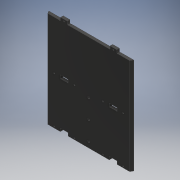
# Autodesk Inventor part: BA04
Saved by Autodesk Inventor 2017 (Build 210142000, 142)
## iProperties
Created: 2019-05-22
Part Number: BA04
Material: Wood (Cherry)
Document SubType Name: Modeling
Designer: Dell
Density: 0.63 g/cm^3
Appearance: Smooth - Black
Mass: 794.992 g
Surface Area: 2256.82 cm^2
Volume: 1261.89 cm^3
Author: Dell
Autodesk Inventor part; units mm, degrees
ref_plane "YZ Plane" through (0, 0, 0) normal (1, 0, 0) x (0, 1, 0)
ref_plane "XZ Plane" through (0, 0, 0) normal (0, 1, 0) x (-1, 0, 0)
ref_plane "XY Plane" through (0, 0, 0) normal (0, 0, 1) x (1, 0, 0)
sketch "Sketch1" plane through (0, 0, 0) normal (0, 0, 1) x (1, 0, 0)
  line L0 (0, 0) -> (303.5592, 0)
  line L1 (303.5592, 0) -> (455.3388, -262.89) construction
  line L2 (455.3388, -262.89) -> (404.5388, -350.8782)
  line L3 (404.5388, -350.8782) -> (-50.8, -87.9882) construction
  line L4 (-50.8, -87.9882) -> (0, 0) construction
  line L5 (0, 0) -> (5.4993, -9.525)
  line L6 (5.4993, -9.525) -> (298.06, -9.525)
  line L7 (298.06, -9.525) -> (303.5592, 0)
  dimension "d0" = 525.78
  dimension "d1" = 101.6
  dimension "d2" = 120
  dimension "d3" = 9.525
  dimension "d4" = 60
  dimension "d5" = 60
  constraints: 16 end point, 2 equal length, 2 horizontal, 2 perpendicular
  measures "d0" distance of L2.end L3.end
  measures "d1" distance of L3.end L0.start
  measures "d2" angle of L0 L4
  measures "d3" distance between parallel lines of L0 L6
  measures "d4" angle of L0 L5
  measures "d5" angle of L0 L7
extrude "Extrusion1" add sketch "Sketch1" along normal blind 342.9
sketch "Sketch2" plane through (5.4993, -9.525, 0) normal (0, -1, 0) x (1, 0, 0)
  line L0 (298.06, 342.9) -> (-5.4993, 342.9) projected
  line L1 (45.3007, 342.9) -> (70.7007, 342.9)
  line L2 (70.7007, 342.9) -> (70.7007, 352.425)
  line L3 (70.7007, 352.425) -> (45.3007, 352.425)
  line L4 (45.3007, 352.425) -> (45.3007, 342.9)
  line L5 (221.86, 342.9) -> (247.26, 342.9)
  line L6 (247.26, 342.9) -> (247.26, 352.425)
  line L7 (247.26, 352.425) -> (221.86, 352.425)
  line L8 (221.86, 352.425) -> (221.86, 342.9)
  line L9 (-5.4993, 0) -> (-5.4993, 342.9) projected
  line L10 (298.06, 0) -> (298.06, 342.9) projected
  circle A0 centre (58.0007, 347.6625) radius 2.25
  circle A1 centre (234.56, 347.6625) radius 2.25
  point P0 (58.0007, 352.425)
  point P1 (234.56, 352.425)
  point P2 (70.7007, 347.6625)
  point P3 (247.26, 347.6625)
  dimension "d8" = 25.4
  dimension "d9" = 9.525
  dimension "d10" = 25.4
  dimension "d11" = 9.525
  dimension "d12" = 50.8
  dimension "d13" = 50.8
  dimension "d16" = 4.5
  dimension "d17" = 4.5
  constraints: 16 end point, 4 midpoint, 4 parallel, 2 centre point, 2 horizontal, 2 horizontal alignment, 2 perpendicular, 2 point on line, 2 vertical alignment
  measures "d8" distance of L3.end L2.end
  measures "d9" distance of L2.end L1.end
  measures "d10" distance of L7.end L6.end
  measures "d11" distance of L6.end L5.end
  measures "d12" distance between parallel lines of L9 L4
  measures "d13" distance between parallel lines of L10 L6
  measures "d16" diameter of A0
  measures "d17" diameter of A1
extrude "Extrusion2" add sketch "Sketch2" against normal blind 9.525
ref_plane "Work Plane1" through (0, 0, 292.1) normal (0, 0, 1) x (1, 0, 0)
sketch "Sketch3" plane through (0, 0, 292.1) normal (0, 0, 1) x (1, 0, 0)
  line L0 (0, 0) -> (303.5592, 0) projected
  line L1 (0, 0) -> (0, -9.525)
  line L2 (298.06, -9.525) -> (5.4993, -9.525) projected
  line L3 (0, -9.525) -> (5.4993, -9.525)
  line L4 (5.4993, -9.525) -> (0, 0) projected
  constraints: 4 end point, 1 perpendicular, 1 vertical
extrude "Extrusion3" [suppressed]
ref_plane "Work Plane2" through (0, 0, 50.8) normal (0, 0, -1) x (-1, 0, 0)
sketch "Sketch4" plane through (0, 0, 50.8) normal (0, 0, -1) x (-1, 0, 0)
  line L0 (0, -12.7) -> (0, 0) projected
  line L1 (-7.3323, -12.7) -> (0, 0) projected
  line L2 (-7.3323, -12.7) -> (0, -12.7) projected
extrude "Extrusion4" [suppressed]
ref_plane "Work Plane3" through (0, 0, 171.45) normal (0, 0, -1) x (-1, 0, 0)
sketch "Sketch5" plane through (0, 0, 171.45) normal (0, 0, -1) x (-1, 0, 0)
  line L0 (0, 0) -> (0, -12.7) projected
  line L1 (0, -12.7) -> (-7.3323, -12.7) projected
  line L2 (0, 0) -> (-7.3323, -12.7) projected
extrude "Extrusion5" [suppressed]
ref_plane "Work Plane4" through (151.7796, -9.525, 342.9) normal (-1, 0, 0) x (0, 0, 1)
mirror "Mirror1" [suppressed]
sketch "Sketch6" plane through (296.2269, -12.7, 292.1) normal (0, 0, 1) x (1, 0, 0)
  line L0 (0, 0) -> (7.3323, 12.7) projected
  line L1 (7.3323, 0) -> (0, 0) projected
  line L2 (7.3323, 12.7) -> (7.3323, 0) projected
  line L3 (7.3323, 12.7) -> (7.3323, 0) projected
  line L4 (0, 0) -> (7.3323, 12.7) projected
  line L5 (7.3323, 0) -> (0, 0) projected
  line L6 (-296.2269, 12.7) -> (-296.2269, 0) projected
  line L7 (-296.2269, 0) -> (-288.8945, 0) projected
  line L8 (-296.2269, 12.7) -> (-288.8945, 0) projected
  line L9 (-296.2269, 0) -> (-296.2269, 12.7) projected
  line L10 (-296.2269, 12.7) -> (-274.2298, 0) construction
  line L11 (0, 0) -> (-288.8945, 0) projected
  line L12 (-285.2269, 6.3491) -> (-285.2269, 0)
  line L13 (-288.8945, 0) -> (-296.2269, 0) projected
  line L14 (-285.2269, 0) -> (-296.2269, 0)
  line L15 (-144.4473, 0) -> (-144.4473, -42.8761)
  line L16 (7.3323, 12.7) -> (7.3323, 0)
  line L17 (7.3323, 0) -> (0, 0)
  line L18 (7.3323, 12.7) -> (0, 0)
  line L19 (7.3323, 0) -> (7.3323, 12.7)
  line L20 (7.3323, 12.7) -> (-14.6647, 0) construction
  line L21 (-3.6677, 6.3491) -> (-3.6677, 0)
  line L22 (0, 0) -> (7.3323, 0)
  line L23 (-3.6677, 0) -> (7.3323, 0)
  line L24 (-288.8945, 0) -> (-296.2269, 12.7) projected
  line L25 (-285.2269, 6.3491) -> (-296.2269, 12.7)
  line L26 (7.3323, 12.7) -> (0, 0) projected
  line L27 (7.3323, 12.7) -> (-3.6677, 6.3491)
  line L28 (0, 0) -> (7.3323, 12.7)
  line L29 (0, 0) -> (-3.6677, 0)
  line L30 (7.3323, 0) -> (7.3323, 12.7) projected
  line L31 (-3.6677, 0) -> (7.3323, 0)
  dimension "d26" = 60
  dimension "d27" = 11
  constraints: 34 end point, 5 symmetric about line, 3 point on line, 2 collinear, 2 horizontal, 1 midpoint, 1 perpendicular, 1 vertical
  measures "d26" angle of L6 L10
  measures "d27" distance between parallel lines of L6 L12
extrude "Extrusion6" [suppressed]
sketch "Sketch7" plane through (0, 0, 184.15) normal (0, 0, 1) x (1, 0, 0)
  line L0 (7.3323, -12.7) -> (0, 0) projected
  line L1 (11, -12.7) -> (7.3323, -12.7) projected
  line L2 (11, -6.3509) -> (11, -12.7) projected
  line L3 (0, 0) -> (11, -6.3509) projected
  line L4 (303.5592, 0) -> (296.2269, -12.7) projected
  line L5 (292.5592, -6.3509) -> (303.5592, 0) projected
  line L6 (292.5592, -12.7) -> (292.5592, -6.3509) projected
  line L7 (296.2269, -12.7) -> (292.5592, -12.7) projected
  line L8 (303.5592, 0) -> (303.5592, -12.7) projected
  line L9 (296.2269, -12.7) -> (303.5592, 0) projected
  line L10 (303.5592, -12.7) -> (296.2269, -12.7) projected
  line L11 (0, 0) -> (0, -12.7) projected
  line L12 (0, -12.7) -> (7.3323, -12.7) projected
  line L13 (0, 0) -> (7.3323, -12.7) projected
extrude "Extrusion7" [suppressed]
sketch "Sketch8" plane through (0, 0, 76.2) normal (0, 0, 1) x (1, 0, 0)
  line L0 (0, 0) -> (0, -12.7) projected
  line L1 (0, -12.7) -> (7.3323, -12.7) projected
  line L2 (0, 0) -> (7.3323, -12.7) projected
  line L3 (7.3323, -12.7) -> (0, 0) projected
  line L4 (11, -12.7) -> (7.3323, -12.7) projected
  line L5 (11, -6.3509) -> (11, -12.7) projected
  line L6 (0, 0) -> (11, -6.3509) projected
  line L7 (303.5592, 0) -> (296.2269, -12.7) projected
  line L8 (292.5592, -6.3509) -> (303.5592, 0) projected
  line L9 (292.5592, -12.7) -> (292.5592, -6.3509) projected
  line L10 (296.2269, -12.7) -> (292.5592, -12.7) projected
  line L11 (303.5592, 0) -> (303.5592, -12.7) projected
  line L12 (296.2269, -12.7) -> (303.5592, 0) projected
  line L13 (303.5592, -12.7) -> (296.2269, -12.7) projected
extrude "Extrusion8" [suppressed]
sketch "Sketch9" plane through (0, 0, 0) normal (0, 0, -1) x (-1, 0, 0)
  line L0 (-251.9796, -9.525) -> (-251.9796, 0)
  line L1 (-251.9796, 0) -> (-226.5796, 0)
  line L2 (-226.5796, 0) -> (-226.5796, -9.525)
  line L3 (-226.5796, -9.525) -> (-251.9796, -9.525)
  line L4 (-76.9796, -9.525) -> (-76.9796, 0)
  line L5 (-76.9796, 0) -> (-51.5796, 0)
  line L6 (-51.5796, 0) -> (-51.5796, -9.525)
  line L7 (-51.5796, -9.525) -> (-76.9796, -9.525)
  line L8 (-239.2796, 0) -> (-64.2796, 0) construction
  circle A0 centre (-239.2796, -4.7625) radius 2.25
  circle A1 centre (-64.2796, -4.7625) radius 2.25
  line L9 (-239.2796, -4.7625) -> (-239.2796, 0) construction
  line L10 (-239.2796, -4.7625) -> (-226.5796, -4.7625) construction
  line L11 (-76.9796, -4.7625) -> (-64.2796, -4.7625) construction
  line L12 (-64.2796, -4.7625) -> (-64.2796, 0) construction
  line L13 (0, 0) -> (-303.5592, 0) projected
  point P0 (-151.7796, 0)
  dimension "d34" = 25.4
  dimension "d35" = 9.525
  dimension "d36" = 9.525
  dimension "d37" = 25.4
  dimension "d38" = 175
  dimension "d39" = 4.5
  dimension "d40" = 4.5
  constraints: 26 end point, 6 midpoint, 6 perpendicular, 4 parallel, 4 point on line, 2 centre point
  measures "d34" distance of L4.end L5.end
  measures "d35" distance of L5.end L7.start
  measures "d36" distance of L0.start L1.start
  measures "d37" distance of L1.start L2.start
  measures "d38" distance of L8.start L12.end
  measures "d39" diameter of A0
  measures "d40" diameter of A1
extrude "Extrusion9" cut sketch "Sketch9" against normal blind 9.525 contours L0 L1 L2 L3 | L4 L5 L6 L7 | A0 | A1
sketch "Sketch10" plane through (227.3592, -9.525, 352.425) normal (0, -1, 0) x (1, 0, 0)
  line L0 (-175.7796, -187.8) -> (-150.3796, -187.8)
  line L1 (-150.3796, -187.8) -> (-150.3796, -178.275)
  line L2 (-150.3796, -178.275) -> (-175.7796, -178.275)
  line L3 (-175.7796, -178.275) -> (-175.7796, -187.8)
  line L4 (-0.7796, -187.8) -> (24.6204, -187.8)
  line L5 (24.6204, -187.8) -> (24.6204, -178.275)
  line L6 (24.6204, -178.275) -> (-0.7796, -178.275)
  line L7 (-0.7796, -178.275) -> (-0.7796, -187.8)
  line L8 (-175.7796, -342.9) -> (-150.3796, -342.9) projected
  line L9 (-0.7796, -342.9) -> (24.6204, -342.9) projected
  line L10 (76.2, -9.525) -> (-227.3592, -9.525) projected
  point P0 (-227.3592, -352.425)
  point P1 (-163.0796, -187.8)
  point P2 (-163.0796, -342.9)
  point P3 (11.9204, -187.8)
  point P4 (11.9204, -342.9)
  point P5 (-176.5592, -9.525)
  dimension "d44" = 25.4
  dimension "d45" = 9.525
  dimension "d46" = 25.4
  dimension "d47" = 9.525
  dimension "d90" = 168.75
  constraints: 16 end point, 4 midpoint, 4 parallel, 2 horizontal, 2 perpendicular, 2 vertical alignment, 1 horizontal alignment
  measures "d44" distance of L2.end L1.end
  measures "d45" distance of L1.end L0.end
  measures "d46" distance of L6.end L5.end
  measures "d47" distance of L5.end L4.end
  measures "d90" distance between parallel lines of L10 L2
extrude "Extrusion10" cut sketch "Sketch10" against normal through all
sketch "Sketch11" plane through (227.3592, -9.525, 352.425) normal (0, -1, 0) x (1, 0, 0)
  line L0 (-150.3796, -352.425) -> (-0.7796, -352.425) construction
  line L1 (-100.9796, -352.425) -> (-50.1796, -352.425) construction
  line L2 (-50.1796, -352.425) -> (-50.1796, -178.275) construction
  line L3 (-50.1796, -178.275) -> (-100.9796, -178.275) construction
  line L4 (-100.9796, -178.275) -> (-100.9796, -352.425) construction
  circle A0 centre (-75.5796, -264.715) radius 4
  circle A1 centre (-75.5796, -197.005) radius 4
  circle A2 centre (-75.5796, -332.425) radius 4
  line L5 (-0.7796, -352.425) -> (-150.3796, -352.425) projected
  circle A3 centre (-198.8198, -183.0375) radius 2.25
  circle A4 centre (-198.8198, -347.6625) radius 2.25
  circle A5 centre (47.6606, -347.6625) radius 2.25
  circle A6 centre (47.6606, -183.0375) radius 2.25
  line L6 (-175.7796, -352.425) -> (-221.86, -352.425) projected
  line L7 (70.7007, -352.425) -> (24.6204, -352.425) projected
  line L8 (-175.7796, -187.8) -> (-175.7796, -178.275) projected
  line L9 (-175.7796, -352.425) -> (-175.7796, -342.9) projected
  line L10 (24.6204, -342.9) -> (24.6204, -352.425) projected
  line L11 (24.6204, -178.275) -> (24.6204, -187.8) projected
  circle A7 centre (-126.3796, -183.0375) radius 2.25
  circle A8 centre (-126.3796, -347.6625) radius 2.25
  circle A9 centre (-24.7796, -347.6625) radius 2.25
  circle A10 centre (-24.7796, -183.0375) radius 2.25
  point P0 (-227.3592, -352.425)
  point P1 (-150.3796, -178.275)
  point P2 (-75.5796, -352.425)
  point P3 (-75.5796, -352.425)
  point P4 (-75.5796, -352.425)
  point P5 (-50.1796, -265.35)
  point P6 (-198.8198, -352.425)
  point P7 (47.6606, -352.425)
  point P8 (-175.7796, -183.0375)
  point P9 (-175.7796, -347.6625)
  point P10 (24.6204, -347.6625)
  point P11 (24.6204, -183.0375)
  point P12 (24.6204, -347.6625)
  dimension "d52" = 8
  dimension "d53" = 8
  dimension "d54" = 8
  dimension "d56" = 20
  dimension "d59" = 50.8
  dimension "d60" = 4.5
  dimension "d61" = 4.5
  dimension "d62" = 4.5
  dimension "d63" = 4.5
  dimension "d64" = 4.5
  dimension "d65" = 4.5
  dimension "d66" = 4.5
  dimension "d67" = 4.5
  dimension "d68" = 25.4
  dimension "d69" = 25.4
  dimension "d96" = 67.71
  dimension "d97" = 67.71
  constraints: 11 centre point, 11 midpoint, 9 horizontal alignment, 9 vertical alignment, 8 end point, 2 parallel, 1 coincident, 1 horizontal, 1 perpendicular, 1 point on line
  measures "d52" diameter of A0
  measures "d53" diameter of A1
  measures "d54" diameter of A2
  measures "d56" distance from line of L0 A2.centre
  measures "d59" distance of L2.end L3.end
  measures "d60" diameter of A3
  measures "d61" diameter of A4
  measures "d62" diameter of A5
  measures "d63" diameter of A6
  measures "d64" diameter of A7
  measures "d65" diameter of A8
  measures "d66" diameter of A9
  measures "d67" diameter of A10
  measures "d68" distance from line of L2 A10.centre
  measures "d69" distance from line of A7.centre L4
  measures "d96" distance of A0.centre A1.centre
  measures "d97" distance of A2.centre A0.centre
extrude "Extrusion11" cut sketch "Sketch11" against normal through all
sketch "Sketch12" plane through (227.3592, -9.525, 352.425) normal (0, -1, 0) x (1, 0, 0)
  line L0 (-175.7796, -352.425) -> (-221.86, -352.425) projected
  line L1 (-177.0496, -352.425) -> (-149.1096, -352.425)
  line L2 (-149.1096, -352.425) -> (-149.1096, -341.63)
  line L3 (-149.1096, -341.63) -> (-177.0496, -341.63)
  line L4 (-177.0496, -341.63) -> (-177.0496, -352.425)
  line L5 (-0.7796, -352.425) -> (-150.3796, -352.425) projected
  line L6 (-2.0496, -352.425) -> (25.8904, -352.425)
  line L7 (25.8904, -352.425) -> (25.8904, -341.63)
  line L8 (25.8904, -341.63) -> (-2.0496, -341.63)
  line L9 (-2.0496, -341.63) -> (-2.0496, -352.425)
  line L10 (-177.0496, -177.005) -> (-149.1096, -177.005)
  line L11 (-149.1096, -177.005) -> (-149.1096, -189.07)
  line L12 (-149.1096, -189.07) -> (-177.0496, -189.07)
  line L13 (-177.0496, -189.07) -> (-177.0496, -177.005)
  line L14 (-2.0496, -177.005) -> (25.8904, -177.005)
  line L15 (25.8904, -177.005) -> (25.8904, -189.07)
  line L16 (25.8904, -189.07) -> (-2.0496, -189.07)
  line L17 (-2.0496, -189.07) -> (-2.0496, -177.005)
  line L18 (-150.3796, -178.275) -> (-150.3796, -187.8) projected
  line L19 (-0.7796, -187.8) -> (-0.7796, -178.275) projected
  line L20 (-175.7796, -178.275) -> (-150.3796, -178.275) projected
  line L21 (-0.7796, -178.275) -> (24.6204, -178.275) projected
  line L22 (-0.7796, -342.9) -> (24.6204, -342.9) projected
  line L23 (-175.7796, -342.9) -> (-150.3796, -342.9) projected
  circle A0 centre (-178.8043, -7.2799) radius 3.175
  circle A1 centre (-148.9142, -7.2799) radius 3.175
  circle A2 centre (-2.2451, -7.2799) radius 3.175
  circle A3 centre (27.6451, -7.2799) radius 3.175
  line L24 (-176.5592, -9.525) -> (-178.8043, -7.2799)
  line L25 (-221.86, -9.525) -> (-176.5592, -9.525) projected
  point P0 (-227.3592, -352.425)
  point P1 (-150.3796, -183.0375)
  point P2 (-149.1096, -183.0375)
  point P3 (-0.7796, -183.0375)
  point P4 (-2.0496, -183.0375)
  point P5 (-163.0796, -178.275)
  point P6 (-163.0796, -177.005)
  point P7 (11.9204, -178.275)
  point P8 (11.9204, -177.005)
  point P9 (11.9204, -342.9)
  point P10 (11.9204, -341.63)
  point P11 (-163.0796, -342.9)
  point P12 (-163.0796, -341.63)
  point P13 (-151.1592, -9.525)
  point P14 (0, -9.525)
  point P15 (25.4, -9.525)
  dimension "d74" = 6.35
  dimension "d75" = 6.35
  dimension "d76" = 6.35
  dimension "d77" = 6.35
  dimension "d70" = 1.27
  dimension "d71" = 1.27
  dimension "d72" = 1.27
  dimension "d73" = 1.27
  dimension "d89" = 45
  constraints: 34 end point, 12 midpoint, 8 parallel, 7 horizontal alignment, 5 vertical alignment, 4 horizontal, 4 perpendicular, 3 point on line, 12 other
  measures "d70" distance between parallel lines of L10 L20
  measures "d71" distance between parallel lines of L17 L19
  measures "d72" distance between parallel lines of L11 L18
  measures "d73" distance between parallel lines of L3 L23
  measures "d89" angle of L25 L24
extrude "Extrusion12" cut sketch "Sketch12" against normal through all
sketch "Sketch13" plane through (227.3592, -9.525, 352.425) normal (0, -1, 0) x (1, 0, 0)
  line L0 (-176.5592, 0) -> (-151.1592, 0)
  line L1 (-151.1592, 0) -> (-151.1592, 1.27)
  line L2 (-151.1592, 1.27) -> (-176.5592, 1.27)
  line L3 (-176.5592, 1.27) -> (-176.5592, 0)
  line L4 (25.4, 0) -> (0, 0)
  line L5 (0, 0) -> (0, 1.27)
  line L6 (0, 1.27) -> (25.4, 1.27)
  line L7 (25.4, 1.27) -> (25.4, 0)
  point P0 (-227.3592, -352.425)
  point P1 (-151.1592, 0)
  dimension "d80" = 1.27
  constraints: 16 end point, 4 parallel, 2 coincident, 2 horizontal, 2 perpendicular, 1 horizontal alignment
  measures "d80" distance of L2.end L0.start
extrude "Extrusion13" add sketch "Sketch13" against normal up to surface (9.525 mm away) from surface at 0
sketch "Sketch14" plane through (298.06, -9.525, 0) normal (0, -1, 0) x (1, 0, 0)
  line L0 (-45.3007, 353.695) -> (-70.7007, 353.695) projected
  line L1 (-45.3007, 353.695) -> (-45.9357, 353.695)
  line L2 (-45.9357, 353.695) -> (-45.9357, 346.4814)
  line L3 (-45.9357, 346.4814) -> (-45.3007, 346.4814)
  line L4 (-45.3007, 346.4814) -> (-45.3007, 353.695)
  arc A0 (-75.1909, 342.9) -> (-70.7007, 347.3901) centre (-72.9458, 345.1451) ccw projected
  line L5 (-70.7007, 353.695) -> (-70.0657, 353.695)
  line L6 (-70.0657, 353.695) -> (-70.0657, 346.4814)
  line L7 (-70.0657, 346.4814) -> (-70.7007, 346.4814)
  line L8 (-70.7007, 346.4814) -> (-70.7007, 353.695)
  arc A1 (-221.86, 347.3901) -> (-217.3698, 342.9) centre (-219.6149, 345.1451) ccw projected
  line L9 (-221.86, 353.695) -> (-222.495, 353.695)
  line L10 (-222.495, 353.695) -> (-222.495, 346.4814)
  line L11 (-222.495, 346.4814) -> (-221.86, 346.4814)
  line L12 (-221.86, 346.4814) -> (-221.86, 353.695)
  line L13 (-247.26, 353.695) -> (-247.26, 347.3901) projected
  line L14 (-247.26, 353.695) -> (-246.625, 353.695)
  line L15 (-246.625, 353.695) -> (-246.625, 346.4814)
  line L16 (-246.625, 346.4814) -> (-247.26, 346.4814)
  line L17 (-247.26, 346.4814) -> (-247.26, 353.695)
  point P0 (-298.06, 0)
  dimension "d91" = 0.635
  dimension "d92" = 0.635
  dimension "d93" = 0.635
  constraints: 32 end point, 8 parallel, 4 horizontal, 4 perpendicular, 3 point on line, 2 point on circle
  measures "d91" distance between parallel lines of L13 L15
  measures "d92" distance between parallel lines of L12 L10
  measures "d93" distance between parallel lines of L4 L2
extrude "Extrusion14" cut sketch "Sketch14" against normal through all
equation "\"d3\" = Panel_Thickness"
equation "\"d9\" = Panel_Thickness"
equation "\"d11\" = Panel_Thickness"
equation "\"d14\" = Panel_Thickness"
equation "\"d35\" = Panel_Thickness"
equation "\"d36\" = Panel_Thickness"
equation "\"d42\" = Panel_Thickness"
equation "\"d45\" = Panel_Thickness"
equation "\"d47\" = Panel_Thickness"
equation "\"d74\" = Tool_Dia"
equation "\"d75\" = Tool_Dia"
equation "\"d76\" = Tool_Dia"
equation "\"d77\" = Tool_Dia"
equation "\"d70\" = Fit_Tolerance"
equation "\"d71\" = Fit_Tolerance"
equation "\"d72\" = Fit_Tolerance"
equation "\"d73\" = Fit_Tolerance"
equation "\"d80\" = Fit_Tolerance"
equation "\"d91\" = 0.5 * Fit_Tolerance"
equation "\"d92\" = 0.5 * Fit_Tolerance"
equation "\"d93\" = 0.5 * Fit_Tolerance"
equation "\"Panel_Thickness\" = 9.525"
equation "\"Fit_Tolerance\" = 1.27"
equation "\"Tool_Dia\" = 6.35"
body "Solid1"
